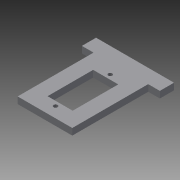
# Autodesk Inventor part: arm-servo
Saved by Autodesk Inventor 2013 (Build 170138000, 138)
## iProperties
Created: 2012-09-08
Part Number: arm-servo
Material: Generic
Document SubType Name: Modeling
Designer: frankenteddy
Density: 1 g/cm^3
Author: frankenteddy
Autodesk Inventor part; units mm, degrees
ref_plane "YZ Plane" through (0, 0, 0) normal (1, 0, 0) x (0, 1, 0)
ref_plane "XZ Plane" through (0, 0, 0) normal (0, 1, 0) x (-1, 0, 0)
ref_plane "XY Plane" through (0, 0, 0) normal (0, 0, 1) x (1, 0, 0)
sketch "Block1" plane through (0, 0, 0) normal (0, 0, 1) x (1, 0, 0)
  circle A0 centre (74.029, 24.2723) radius 1
  line L0 (49.279, 30.4723) -> (71.779, 30.4723)
  line L1 (71.779, 30.4723) -> (71.779, 18.0723)
  line L2 (71.779, 18.0723) -> (49.279, 18.0723)
  line L3 (49.279, 18.0723) -> (49.279, 30.4723)
  line L4 (49.279, 30.4723) -> (44.779, 30.4723)
  line L5 (44.779, 30.4723) -> (44.779, 18.0723)
  line L6 (44.779, 18.0723) -> (49.279, 18.0723)
  line L7 (49.279, 18.0723) -> (49.279, 30.4723)
  line L8 (71.779, 30.4723) -> (76.279, 30.4723)
  line L9 (76.279, 30.4723) -> (76.279, 18.0723)
  line L10 (76.279, 18.0723) -> (71.779, 18.0723)
  line L11 (71.779, 18.0723) -> (71.779, 30.4723)
  line L12 (44.779, 24.2723) -> (76.279, 24.2723) construction
  line L13 (47.029, 30.4723) -> (47.029, 18.0723) construction
  circle A1 centre (47.029, 24.2723) radius 1
  line L14 (74.029, 30.4723) -> (74.029, 18.0723) construction
  point P0 (60.979, 24.0984)
  dimension "d7" = 22.5
  dimension "d8" = 12.4
  dimension "d9" = 4.5
  dimension "d10" = 4.5
  dimension "d11" = 2
  dimension "d12" = 2
  measures "d7" distance of L1.end L2.end
  measures "d8" distance of L0.end L1.end
  measures "d9" distance of L6.end L5.end
  measures "d10" distance of L9.end L10.end
  measures "d11" diameter of A0
  measures "d12" diameter of A1
sketch "Sketch1" plane through (0, 0, 0) normal (0, 0, 1) x (1, 0, 0)
  line L0 (-54.534, 30.732) -> (-16.034, 30.732)
  line L1 (-16.034, 30.732) -> (-16.034, 23.732)
  line L2 (-16.034, 23.732) -> (-54.534, 23.732)
  line L3 (-54.534, 23.732) -> (-54.534, 30.732)
  line L4 (-92.7646, -8.503) -> (-89.7646, -8.503)
  line L5 (-89.7646, -8.503) -> (-89.7646, -11.753)
  line L6 (-89.7646, -11.753) -> (-92.7646, -11.753)
  line L7 (-92.7646, -11.753) -> (-92.7646, -8.503)
  line L8 (-92.7646, -21.6527) -> (-89.7646, -21.6527)
  line L9 (-89.7646, -21.6527) -> (-89.7646, -21.7527)
  line L10 (-89.7646, -21.7527) -> (-92.7646, -21.7527)
  line L11 (-92.7646, -21.7527) -> (-92.7646, -21.6527)
  line L12 (-48.784, 23.732) -> (-21.784, 23.732)
  line L13 (-21.784, 23.732) -> (-21.784, -13.768)
  line L14 (-21.784, -13.768) -> (-48.784, -13.768)
  line L15 (-48.784, -13.768) -> (-48.784, 23.732)
  line L16 (-35.284, 30.732) -> (-35.284, 23.732) construction
  line L17 (-35.284, -13.768) -> (-35.284, 23.732) construction
  circle A0 centre (-35.284, 18.482) radius 1
  line L18 (-41.484, -6.268) -> (-41.484, 16.232)
  line L19 (-41.484, 16.232) -> (-29.084, 16.232)
  line L20 (-29.084, 16.232) -> (-29.084, -6.268)
  line L21 (-29.084, -6.268) -> (-41.484, -6.268)
  line L22 (-41.484, -6.268) -> (-41.484, -10.768)
  line L23 (-41.484, -10.768) -> (-29.084, -10.768)
  line L24 (-29.084, -10.768) -> (-29.084, -6.268)
  line L25 (-29.084, -6.268) -> (-41.484, -6.268)
  line L26 (-41.484, 16.232) -> (-41.484, 20.732)
  line L27 (-41.484, 20.732) -> (-29.084, 20.732)
  line L28 (-29.084, 20.732) -> (-29.084, 16.232)
  line L29 (-29.084, 16.232) -> (-41.484, 16.232)
  line L30 (-35.284, -10.768) -> (-35.284, 20.732) construction
  line L31 (-41.484, -8.518) -> (-29.084, -8.518) construction
  circle A1 centre (-35.284, -8.518) radius 1
  line L32 (-41.484, 18.482) -> (-29.084, 18.482) construction
  point P0 (0, 0)
  dimension "d0" = 3
  dimension "mat" = 3.25
  dimension "d2" = 3
  dimension "d3" = 0.1
  dimension "d4" = 38.5
  dimension "d6" = 7
  dimension "d15" = 3
  dimension "d17" = 27
  dimension "d19" = 3
  dimension "d20" = 37.5
  constraints: 36 end point, 8 parallel, 4 midpoint, 4 perpendicular, 3 horizontal, 1 collinear, 1 point on line, 1 vertical
  measures "d0" distance of L5.end L7.start
  measures "mat" distance of L5.start L5.end
  measures "d2" distance of L9.end L11.start
  measures "d3" distance of L9.start L9.end
  measures "d4" distance of L1.end L2.end
  measures "d6" distance of L0.end L1.end
  measures "d17" distance of L13.end L14.end
  measures "d20" distance of L12.end L13.end
extrude "Extrusion1" add sketch "Sketch1" along normal blind 3.25 contours L0 L1 L2 L3 | L2 L13 L14 L15 | L21 L24 L23 L22 | L26 L27 L28 L19
equation "\"d21\" = mat"
body "Solid1"
